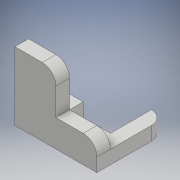
# Autodesk Inventor part: 5
Saved by Autodesk Inventor 2017 (Build 210142000, 142)
## iProperties
Part Number: 5
Material: 一般
Document SubType Name: Modeling
Designer: Brian
Density: 1 g/cm^3
Appearance: 預設
Author: Brian
Autodesk Inventor part; units mm, degrees
ref_plane "YZ Plane" through (0, 0, 0) normal (1, 0, 0) x (0, 1, 0)
ref_plane "XZ Plane" through (0, 0, 0) normal (0, 1, 0) x (-1, 0, 0)
ref_plane "XY Plane" through (0, 0, 0) normal (0, 0, 1) x (1, 0, 0)
sketch "草圖1" plane through (0, 0, 0) normal (0, 1, 0) x (-1, 0, 0)
  line L0 (0, 0) -> (-30, 0)
  line L1 (-30, 0) -> (-30, -50)
  line L2 (-30, -50) -> (0, -50)
  line L3 (0, -50) -> (0, 0)
  line L4 (-30, -50) -> (-60, -50)
  line L5 (-60, -50) -> (-60, -30)
  line L6 (-60, -30) -> (-30, -30)
  line L7 (-30, -30) -> (-30, -50)
  dimension "d0" = 30
  dimension "d1" = 20
  dimension "d2" = 30
  dimension "d6" = 30
  constraints: 16 end point, 4 parallel, 2 horizontal, 2 perpendicular
  measures "d0" distance of L0.start L0.end
  measures "d1" distance of L4.end L5.end
  measures "d2" distance of L5.end L6.end
  measures "d6" distance between parallel lines of L0 L6
extrude "擠出1" add sketch "草圖1" along normal blind 10
sketch "草圖2" plane through (60, 0, -50) normal (0, 0, -1) x (-1, 0, 0)
  line L0 (60, 0) -> (60, 10) projected
  line L1 (60, 10) -> (40, 10)
  line L2 (40, 10) -> (40, 30)
  line L3 (40, 30) -> (60, 30)
  line L4 (60, 30) -> (60, 10)
  line L5 (40, 10) -> (10, 10)
  line L6 (10, 10) -> (10, 20)
  line L7 (10, 20) -> (40, 20)
  line L8 (40, 20) -> (40, 10)
  line L9 (10, 10) -> (0, 10)
  line L10 (0, 10) -> (0, 50)
  line L11 (0, 50) -> (10, 50)
  line L12 (10, 50) -> (10, 10)
  dimension "d7" = 10
  dimension "d8" = 30
  dimension "d9" = 20
  dimension "d10" = 20
  dimension "d11" = 10
  dimension "d12" = 40
  constraints: 24 end point, 6 parallel, 3 horizontal, 3 perpendicular
  measures "d7" distance of L10.end L11.end
  measures "d8" distance of L6.end L7.end
  measures "d9" distance of L2.end L3.end
  measures "d10" distance of L3.end L0.end
  measures "d11" distance between parallel lines of L5 L7
  measures "d12" distance of L9.end L10.end
extrude "擠出2" add sketch "草圖2" against normal blind 10
sketch "草圖3" plane through (0, 0, -50) normal (-1, 0, 0) x (0, 0, 1)
  line L0 (0, 30) -> (10, 30) projected
  line L1 (50, 10) -> (20, 10) projected
  line L2 (10, 30) -> (50, 10)
  line L3 (50, 10) -> (10, 10)
  line L4 (10, 20) -> (10, 30) projected
  line L5 (10, 10) -> (10, 30)
  point P0 (50, 0)
  constraints: 6 end point, 1 collinear, 1 perpendicular
extrude "擠出3" add sketch "草圖3" against normal blind 10
fillet "圓角1" radius 10 3 edges at (60, 50, -45) (60, 5, -30) (30, 5, 0)
